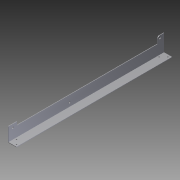
# Autodesk Inventor part: 8 ball top roller L frame
Saved by Autodesk Inventor 2012 (Build 160160000, 160)
## iProperties
Created: 2013-10-29
Part Number: 8 ball top roller L frame
Material: Default
Document SubType Name: Modeling
Designer: Bryce
Density: 1 g/cm^3
Author: Bryce
Autodesk Inventor part; units mm, degrees
ref_plane "YZ Plane" through (0, 0, 0) normal (1, 0, 0) x (0, 1, 0)
ref_plane "XZ Plane" through (0, 0, 0) normal (0, 1, 0) x (-1, 0, 0)
ref_plane "XY Plane" through (0, 0, 0) normal (0, 0, 1) x (1, 0, 0)
sketch "Sketch1" plane through (0, 0, 0) normal (0, 0, 1) x (1, 0, 0)
  line L0 (0, 0) -> (25.4, 0)
  line L1 (25.4, 0) -> (25.4, 1.5875)
  line L2 (1.5875, 50.8) -> (0, 50.8)
  line L3 (0, 50.8) -> (0, 0)
  line L4 (1.5875, 50.8) -> (1.5875, 1.5875)
  line L5 (1.5875, 1.5875) -> (25.4, 1.5875)
  dimension "d0" = 1.5875
  dimension "d1" = 1.5875
  dimension "d2" = 25.4
  dimension "d3" = 50.8
  constraints: 12 end point, 2 parallel, 1 horizontal, 1 perpendicular
  measures "d0" distance between parallel lines of L4 L3
  measures "d1" distance between parallel lines of L0 L5
  measures "d2" distance of L0.start L0.end
  measures "d3" distance of L2.end L0.start
extrude "Extrusion1" add sketch "Sketch1" along normal blind 457.2
sketch "Sketch2" plane through (0, 0, 0) normal (-1, 0, 0) x (0, 0, 1)
  line L0 (457.2, 0) -> (457.2, 50.8) projected
  line L1 (0, 50.8) -> (457.2, 50.8) projected
  line L2 (0, 50.8) -> (0, 0) projected
  line L3 (0, 0) -> (457.2, 0) projected
  line L4 (19.05, 50.8) -> (19.05, 31.75)
  line L5 (19.05, 31.75) -> (431.8, 31.75)
  circle A0 centre (12.7, 44.45) radius 3.175
  arc A1 (19.05, 44.45) -> (12.7, 50.8) centre (12.7, 44.45) ccw
  circle A2 centre (444.5, 31.75) radius 11.1125 construction
  line L6 (431.8, 31.75) -> (431.8, 41.275)
  circle A3 centre (444.5, 31.75) radius 2.54
  line L7 (431.8, 41.275) -> (457.2, 41.275)
  circle A4 centre (277.8125, 12.7) radius 11.1125 construction
  circle A5 centre (277.8125, 12.7) radius 2.54
  line L8 (266.7, 0) -> (266.7, -29.1939)
  dimension "d6" = 19.05
  dimension "d7" = 19.05
  dimension "d8" = 6.35
  dimension "d9" = 12.7
  dimension "d10" = 6.35
  dimension "d13" = 22.225
  dimension "d14" = 25.4
  dimension "d15" = 5.08
  dimension "d16" = 31.75
  dimension "d17" = 12.7
  dimension "d18" = 9.525
  dimension "d19" = 12.7
  dimension "d27" = 190.5
  constraints: 10 end point, 6 centre point, 5 perpendicular, 5 point on line, 3 coincident, 2 equal radius, 2 point on circle, 2 tangent
  measures "d6" distance between parallel lines of L4 L2
  measures "d7" distance of L4.start L4.end
  measures "d8" diameter of A0
  measures "d9" distance from line of L2 A0.centre
  measures "d10" distance from line of L1 A0.centre
  measures "d13" diameter of A2
  measures "d14" distance between parallel lines of L0 L6
  measures "d15" diameter of A3
  measures "d16" distance from line of L3 A3.centre
  measures "d17" distance from line of L0 A2.centre
  measures "d18" distance of L5.end L6.end
  measures "d19" distance from line of L3 A4.centre
  measures "d27" distance between parallel lines of L0 L8
extrude "Extrusion2" cut sketch "Sketch2" against normal through all contours L7 L6 L5 L4 L1 L0 | L4 A1 L1 | A0 | A3 | A5
sketch "Sketch3" plane through (0, 0, 0) normal (0, -1, 0) x (1, 0, 0)
  line L0 (0, 0) -> (0, 457.2) projected
  line L1 (0, 0) -> (25.4, 0) projected
  line L2 (25.4, 0) -> (25.4, 457.2) projected
  circle A0 centre (19.05, 6.35) radius 1.5875
  circle A1 centre (6.35, 19.05) radius 1.5875
  line L3 (0, 228.6) -> (25.4, 228.6) construction
  circle A2 centre (19.05, 450.85) radius 1.5875
  circle A3 centre (6.35, 438.15) radius 1.5875
  dimension "d20" = 3.175
  dimension "d21" = 6.35
  dimension "d22" = 6.35
  dimension "d23" = 19.05
  dimension "d24" = 6.35
  constraints: 4 centre point, 2 end point, 2 midpoint, 2 symmetric about line, 1 equal radius, 2 other
  measures "d20" diameter of A1
  measures "d21" distance from line of L2 A0.centre
  measures "d22" distance from line of L0 A1.centre
  measures "d23" distance from line of L1 A1.centre
  measures "d24" distance from line of A0.centre L1
extrude "Extrusion3" cut sketch "Sketch3" against normal through all
equation "\"d0\" = d1"
equation "\"d21\" = d22"
equation "\"d24\" = d21"
body "Solid1"
